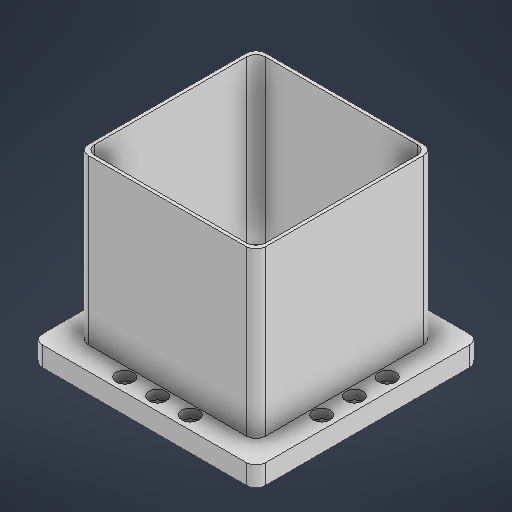
# Autodesk Inventor part: Shield
Saved by Autodesk Inventor 2025 (Build 290162000, 162)
## iProperties
Created: 2025-08-15
Part Number: Shield
Material: Generic
Document SubType Name: Modeling
Designer: mayhem
Density: 1 g/cm^3
Appearance: Default
Author: mayhem
Autodesk Inventor part; units mm, degrees
ref_plane "YZ Plane" through (0, 0, 0) normal (1, 0, 0) x (0, 1, 0)
ref_plane "XZ Plane" through (0, 0, 0) normal (0, 1, 0) x (-1, 0, 0)
ref_plane "XY Plane" through (0, 0, 0) normal (0, 0, 1) x (1, 0, 0)
sketch "Sketch1" plane through (0, 0, 0) normal (0, 1, 0) x (-1, 0, 0)
  line L0 (85, 85) -> (-85, 85)
  line L1 (-85, 85) -> (-85, -85)
  line L2 (-85, -85) -> (85, -85)
  line L3 (85, -85) -> (85, 85)
  line L4 (47, -65) -> (-47, -65)
  line L5 (-65, -47) -> (-65, 47)
  line L6 (-47, 65) -> (47, 65)
  line L7 (65, 47) -> (65, -47)
  line L8 (0, 0) -> (0, 20)
  line L9 (0, 0) -> (15.875, 0)
  arc A0 (-65, -63) -> (-63, -65) centre (-63, -63) ccw
  arc A1 (-65, -47) -> (-47, -65) centre (-47, -47) ccw
  arc A2 (47, -65) -> (65, -47) centre (47, -47) ccw
  arc A3 (65, 47) -> (47, 65) centre (47, 47) ccw
  arc A4 (-47, 65) -> (-65, 47) centre (-47, 47) ccw
  point P0 (65, -65)
  point P1 (-65, -65)
  point P2 (-65, 65)
  point P3 (65, 65)
  point P4 (-65, -45)
  point P5 (-45, -65)
  point P6 (-65, 0)
  point P7 (0, -65)
  dimension "d50" = 45
  dimension "d51" = 170
  dimension "d52" = 170
  dimension "d53" = 20
  dimension "d54" = 130
  dimension "d55" = 130
  dimension "d56" = 45
  dimension "d62" = 2
  dimension "d63" = 20
  dimension "d64" = 18
  constraints: 20 end point, 12 point on line, 10 point on circle, 10 tangent, 5 centre point, 4 parallel, 3 equal radius, 2 midpoint, 2 perpendicular, 1 horizontal, 1 vertical
  measures "d50" distance of point (-65, 0) point (-65, -45)
  measures "d51" distance of L2.end L0.start
  measures "d52" distance of L1.end L2.end
  measures "d53" distance between parallel lines of L2 L4
  measures "d54" distance of point (65, 65) point (65, -65)
  measures "d55" distance of point (65, -65) point (-65, -65)
  measures "d56" distance of point (0, -65) point (-45, -65)
  measures "d62" radius of A0
  measures "d63" distance between parallel lines of L5 L1
  measures "d64" radius of A1
extrude "Extrusion1" add sketch "Sketch1" along normal blind 15
sketch "Sketch3" plane through (0, 15, 0) normal (0, 1, 0) x (1, 0, 0)
  line L0 (-75, 75) -> (75, 75)
  line L1 (75, 75) -> (75, -75)
  line L2 (75, -75) -> (-75, -75)
  line L3 (-75, -75) -> (-75, 75)
  line L4 (-75, 75) -> (75, -75) construction
  line L5 (75, 75) -> (-75, -75) construction
  circle A0 centre (0, -75) radius 3
  circle A1 centre (-25, -75) radius 3
  circle A2 centre (25, -75) radius 3
  circle A3 centre (75, 0) radius 3
  circle A4 centre (75, 25) radius 3
  circle A5 centre (75, -25) radius 3
  circle A6 centre (-75, 0) radius 3
  circle A7 centre (-75, -25) radius 3
  circle A8 centre (-75, 25) radius 3
  circle A9 centre (0, 75) radius 3
  circle A10 centre (25, 75) radius 3
  circle A11 centre (-25, 75) radius 3
  point P0 (0, 0)
  dimension "d30" = 150
  dimension "d31" = 150
  dimension "d32" = 6
  dimension "d33" = 6
  dimension "d34" = 6
  dimension "d35" = 6
  dimension "d36" = 6
  dimension "d37" = 6
  dimension "d38" = 25
  dimension "d39" = 25
  dimension "d40" = 25
  dimension "d41" = 25
  constraints: 12 centre point, 12 end point, 6 symmetric about line, 4 midpoint, 4 point on line, 2 parallel, 1 horizontal, 1 perpendicular, 6 other
  measures "d30" distance of L1.end L2.end
  measures "d31" distance of L0.end L1.end
  measures "d32" diameter of A0
  measures "d33" diameter of A1
  measures "d34" diameter of A2
  measures "d35" diameter of A3
  measures "d36" diameter of A4
  measures "d37" diameter of A5
  measures "d38" distance of A2.centre A0.centre
  measures "d39" distance of A0.centre A1.centre
  measures "d40" distance of A3.centre A5.centre
  measures "d41" distance of A3.centre A4.centre
hole "Hole1" at (-25, 15, 75) at (0, 15, 75) at (25, 15, 75) at (75, 15, 25) at (75, 15, 0) at (75, 15, -25) at (25, 15, -75) at (0, 15, -75) at (-25, 15, -75) at (-75, 15, -25) at (-75, 15, 0) at (-75, 15, 25) direction (0, -1, 0) diameter 7.125 end through all counterbore diameter 13 counterbore depth 7
sketch "Sketch4" plane through (0, 15, 0) normal (0, 1, 0) x (1, 0, 0)
  line L0 (65, 65) -> (-65, 65)
  line L1 (-65, 65) -> (-65, -65)
  line L2 (-65, -65) -> (65, -65)
  line L3 (65, -65) -> (65, 65)
  line L4 (65, 65) -> (-65, -65) construction
  line L5 (-65, 65) -> (65, -65) construction
  line L6 (-67.5, 67.5) -> (67.5, 67.5)
  line L7 (67.5, 67.5) -> (67.5, -67.5)
  line L8 (67.5, -67.5) -> (-67.5, -67.5)
  line L9 (-67.5, -67.5) -> (-67.5, 67.5)
  point P0 (0, 0)
  dimension "d57" = 130
  dimension "d58" = 130
  dimension "d59" = 2.5
  constraints: 20 end point, 4 parallel, 2 midpoint, 2 perpendicular, 1 horizontal, 3 other
  measures "d57" distance of L2.end L1.end
  measures "d58" distance between parallel lines of L0 L2
  measures "d59" distance between parallel lines of L0 L6
extrude "Extrusion3" add sketch "Sketch4" along normal blind 125
fillet "Fillet2" radius 7.125 12 edges at (65, 77.5, 65) (67.5, 77.5, 67.5) (-67.5, 77.5, 67.5) (-65, 77.5, 65) (-65, 77.5, -65) (-67.5, 77.5, -67.5) (67.5, 77.5, -67.5) (65, 77.5, -65) (-85, 7.5, 85) (85, 7.5, 85) (85, 7.5, -85) (-85, 7.5, -85)
body "Solid1"
